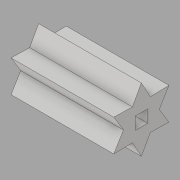
# Autodesk Inventor part: starLatch
Saved by Autodesk Inventor 2017 (Build 210142000, 142)
## iProperties
Created: 2019-05-14
Part Number: starLatch
Material: Generic
Document SubType Name: Modeling
Designer: Joe Sedutto
Density: 1 g/cm^3
Appearance: Default
Author: Joe Sedutto
Autodesk Inventor part; units mm, degrees
ref_plane "YZ Plane" through (0, 0, 0) normal (1, 0, 0) x (0, 1, 0)
ref_plane "XZ Plane" through (0, 0, 0) normal (0, 1, 0) x (-1, 0, 0)
ref_plane "XY Plane" through (0, 0, 0) normal (0, 0, 1) x (1, 0, 0)
sketch "Sketch1" plane through (0, 0, 0) normal (1, 0, 0) x (0, 1, 0)
  line L0 (0, 0) -> (3.048, 0)
  line L1 (3.048, 0) -> (3.048, -3.048)
  line L2 (3.048, -3.048) -> (0, -3.048)
  line L3 (0, -3.048) -> (0, 0)
  line L4 (1.524, -1.524) -> (1.524, -3.048) construction
  line L5 (1.524, -1.524) -> (0, -1.524) construction
  line L6 (4.318, -4.318) -> (4.318, 1.27)
  line L7 (4.318, 1.27) -> (-1.27, 1.27)
  line L8 (-1.27, 1.27) -> (-1.27, -4.318)
  line L9 (-1.27, -4.318) -> (4.318, -4.318)
  line L10 (4.318, 1.27) -> (9.398, -1.524)
  line L11 (9.398, -1.524) -> (4.318, -4.318)
  line L12 (0.5013, 2.2927) -> (5.461, 5.2951)
  line L13 (5.461, 5.2951) -> (5.3407, -0.5013)
  line L14 (5.3407, -0.5013) -> (0.5013, 2.2927)
  line L15 (-2.2927, -0.5013) -> (-2.413, 5.2951)
  line L16 (-2.413, 5.2951) -> (2.5467, 2.2927)
  line L17 (2.5467, 2.2927) -> (-2.2927, -0.5013)
  line L18 (-1.27, -4.318) -> (-6.35, -1.524)
  line L19 (-6.35, -1.524) -> (-1.27, 1.27)
  line L20 (-1.27, 1.27) -> (-1.27, -4.318)
  line L21 (2.5467, -5.3407) -> (-2.413, -8.3431)
  line L22 (-2.413, -8.3431) -> (-2.2927, -2.5467)
  line L23 (-2.2927, -2.5467) -> (2.5467, -5.3407)
  line L24 (5.3407, -2.5467) -> (5.461, -8.3431)
  line L25 (5.461, -8.3431) -> (0.5013, -5.3407)
  line L26 (0.5013, -5.3407) -> (5.3407, -2.5467)
  dimension "d0" = 3.048
  dimension "d1" = 1.27
  dimension "d2" = 5.08
  dimension "d5" = 360
  constraints: 54 end point, 4 parallel, 4 perpendicular, 2 equal length, 2 midpoint, 1 horizontal, 40 other
  measures "d0" distance of L1.end L2.end
  measures "d1" distance between parallel lines of L1 L6
  measures "d2" distance from line of L6 L10.end
extrude "Extrusion1" add sketch "Sketch1" along normal blind 25.4 contours L9 L26 L6 | L11 L24 L25 L21 L23 L26 L9 | L6 L26 L24 L11 | L26 L9 L23 L8 L17 L7 L14 L6 | L6 L14 L13 L10 L11 L24 L26 | L14 L7 L6 | L6 L10 L13 L14 | L23 L26 L25 L21 L22 L18 L9 | L9 L8 L23 | L23 L21 L25 L26 | L7 L14 L17 L16 L12 L13 L10 | L18 L22 L23 L8 | L23 L22 L18 L19 L15 L17 L8 | L17 L8 L7 | L7 L19 L15 L16 L12 L14 L17 | L14 L12 L16 L17 | L17 L15 L19 L8
sketch "Sketch2" plane through (25.4, 0, 0) normal (1, 0, 0) x (0, 0, -1)
  line L0 (-1.7022, 1.524) -> (-1.27, 2.2727) projected
  line L1 (-1.27, 2.2727) -> (-1.27, 0.7753) projected
  line L2 (-1.27, 0.7753) -> (-1.7022, 1.524) projected
  line L3 (3.7419, -2.3175) -> (8.3431, -2.413) projected
  line L4 (8.3431, -2.413) -> (5.9598, 1.524) projected
  line L5 (5.9598, 1.524) -> (8.3431, 5.461) projected
  line L6 (8.3431, 5.461) -> (3.7419, 5.3655) projected
  line L7 (3.7419, 5.3655) -> (1.524, 9.398) projected
  line L8 (1.524, 9.398) -> (-0.6939, 5.3655) projected
  line L9 (-0.6939, 5.3655) -> (-5.2951, 5.461) projected
  line L10 (-5.2951, 5.461) -> (-2.9118, 1.524) projected
  line L11 (-2.9118, 1.524) -> (-5.2951, -2.413) projected
  line L12 (-5.2951, -2.413) -> (-0.6939, -2.3175) projected
  line L13 (-0.6939, -2.3175) -> (1.524, -6.35) projected
  line L14 (1.524, -6.35) -> (3.7419, -2.3175) projected
  line L15 (0, 3.048) -> (3.048, 3.048) projected
  line L16 (3.048, 3.048) -> (3.048, 0) projected
  line L17 (3.048, 0) -> (0, 0) projected
  line L18 (0, 0) -> (0, 3.048) projected
  line L19 (4.7502, 1.524) -> (4.318, 0.7753) projected
  line L20 (4.318, 0.7753) -> (4.318, 2.2727) projected
  line L21 (4.318, 2.2727) -> (4.7502, 1.524) projected
extrude "Extrusion2" add sketch "Sketch2" against normal blind 25.4 contours L0 L1 L2 | L14 L13 L12 L11 L10 L9 L8 L7 L6 L5 L4 L3 | L19 L20 L21
body "Solid1"
